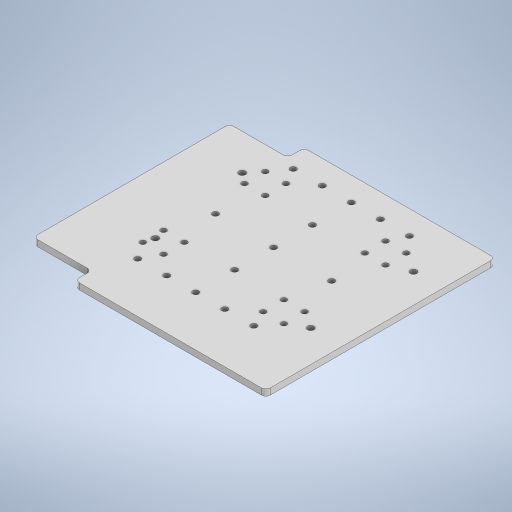
# Autodesk Inventor part: фанера
Saved by Autodesk Inventor 2023 (Build 270158000, 158)
## iProperties
Created: 2025-01-21
Part Number: фанера
Material: Типовые
Document SubType Name: Modeling
Designer: DELL
Density: 1 g/cm^3
Appearance: По умолчанию
Author: DELL
Autodesk Inventor part; units mm, degrees
ref_plane "YZ Plane" through (0, 0, 0) normal (1, 0, 0) x (0, 1, 0)
ref_plane "XZ Plane" through (0, 0, 0) normal (0, 1, 0) x (-1, 0, 0)
ref_plane "XY Plane" through (0, 0, 0) normal (0, 0, 1) x (1, 0, 0)
sketch "Эскиз1" plane through (0, 0, 0) normal (0, 1, 0) x (-1, 0, 0)
  line L0 (-60, 55.25) -> (60, 55.25)
  line L1 (60, 55.25) -> (60, -55.25)
  line L2 (60, -55.25) -> (-60, -55.25)
  line L3 (-60, -55.25) -> (-60, 55.25)
  line L4 (60, -55.25) -> (-60, 55.25) construction
  point P0 (0, 0)
  point P1 (0, 0)
  dimension "d0" = 120
  dimension "d1" = 110.5
  constraints: 10 end point, 2 parallel, 1 coincident, 1 horizontal, 1 midpoint, 1 perpendicular
  measures "d0" distance of L1.end L2.end
  measures "d1" distance of L2.end L0.start
extrude "Выдавливание1" add sketch "Эскиз1" along normal blind 3
sketch "Эскиз2" plane through (0, 3, 0) normal (0, 1, 0) x (1, 0, 0)
  line L0 (-60, 55.25) -> (60, 55.25) projected
  line L1 (-60, 55.25) -> (-32, 55.25)
  line L2 (-32, 55.25) -> (-32, 47.25)
  line L3 (-32, 47.25) -> (-60, 47.25)
  line L4 (-60, 47.25) -> (-60, 55.25)
  line L5 (-60, -55.25) -> (-60, 55.25) projected
  line L6 (-60, -55.25) -> (-32, -55.25)
  line L7 (-32, -55.25) -> (-32, -47.25)
  line L8 (-32, -47.25) -> (-60, -47.25)
  line L9 (-60, -47.25) -> (-60, -55.25)
  point P0 (-60, -47.25)
  dimension "d12" = 28
  dimension "d13" = 8
  dimension "d14" = 28
  dimension "d15" = 8
  constraints: 16 end point, 4 parallel, 2 horizontal, 2 perpendicular
  measures "d12" distance of L2.end L3.end
  measures "d13" distance of L1.end L2.end
  measures "d14" distance of L8.end L7.end
  measures "d15" distance of L7.end L6.end
extrude "Выдавливание2" cut sketch "Эскиз2" against normal blind 10
fillet "Сопряжение2" radius 2 8 edges at (-60, 1.5, 47.25) (-32, 1.5, 47.25) (-32, 1.5, 55.25) (-60, 1.5, -47.25) (-32, 1.5, -47.25) (-32, 1.5, -55.25) (60, 1.5, -55.25) (60, 1.5, 55.25)
sketch "Эскиз3" plane through (0, 3, 0) normal (0, 1, 0) x (1, 0, 0)
  circle A0 centre (-21.5, -13.0622) radius 1.35 projected
  circle A1 centre (-21.5, 35.9378) radius 1.35 projected
  circle A2 centre (36.5, 35.9378) radius 1.35 projected
  circle A3 centre (36.5, -13.0622) radius 1.35 projected
  line L0 (36.5, 25.9378) -> (-21.5, 25.9378) construction
  line L1 (-21.5, 25.9378) -> (-21.5, -23.0622) construction
  line L2 (-21.5, -23.0622) -> (36.5, -23.0622) construction
  line L3 (36.5, -23.0622) -> (36.5, 25.9378) construction
  circle A4 centre (36.5, -23.0622) radius 1.35
  circle A5 centre (36.5, 25.9378) radius 1.35
  circle A6 centre (-21.5, 25.9378) radius 1.35
  circle A7 centre (-21.5, -23.0622) radius 1.35
  line L4 (26.5, 35.9378) -> (-31.5, 35.9378) construction
  line L5 (-31.5, 35.9378) -> (-31.5, -13.0622) construction
  line L6 (-31.5, -13.0622) -> (26.5, -13.0622) construction
  line L7 (26.5, -13.0622) -> (26.5, 35.9378) construction
  circle A8 centre (-31.5, 35.9378) radius 1.35
  circle A9 centre (-31.5, -13.0622) radius 1.35
  circle A10 centre (26.5, -13.0622) radius 1.35
  circle A11 centre (26.5, 35.9378) radius 1.35
  line L8 (26.5, -23.0622) -> (-31.5, -23.0622) construction
  line L9 (-31.5, -23.0622) -> (-31.5, 25.9378) construction
  line L10 (-31.5, 25.9378) -> (26.5, 25.9378)
  line L11 (26.5, 25.9378) -> (26.5, -23.0622) construction
  circle A12 centre (26.5, 25.9378) radius 1.35
  circle A13 centre (26.5, -23.0622) radius 1.35
  circle A14 centre (-31.5, 25.9378) radius 1.35
  circle A15 centre (-31.5, -23.0622) radius 1.35
  point P0 (0, 0)
  dimension "d17" = 58
  dimension "d18" = 49
  dimension "d19" = 10
  dimension "d20" = 58
  dimension "d21" = 49
  dimension "d22" = 10
  dimension "d23" = 2.7
  dimension "d24" = 2.7
  dimension "d25" = 2.7
  dimension "d27" = 58
  dimension "d28" = 49
  dimension "d29" = 2.7
  dimension "d30" = 2.7
  dimension "d31" = 2.7
  dimension "d32" = 2.7
  constraints: 24 end point, 12 centre point, 12 coincident, 6 parallel, 3 horizontal, 3 perpendicular, 2 point on line
  measures "d17" distance of L2.end L1.end
  measures "d18" distance of L1.end L0.end
  measures "d19" distance from line of L0 A2.centre
  measures "d20" distance of L6.end L5.end
  measures "d21" distance of L5.end L4.end
  measures "d22" distance from line of A2.centre L7
  measures "d23" diameter of A8
  measures "d24" diameter of A10
  measures "d25" diameter of A11
  measures "d27" distance of L9.end L10.end
  measures "d28" distance of L8.end L9.end
  measures "d29" diameter of A12
  measures "d30" diameter of A13
  measures "d31" diameter of A14
  measures "d32" diameter of A15
extrude "Выдавливание3" cut sketch "Эскиз3" against normal blind 10
sketch "Эскиз4" plane through (0, 3, 0) normal (0, 1, 0) x (1, 0, 0)
  circle A0 centre (-30.17, -18.3745) radius 1.5875
  circle A1 centre (-36.52, 29.8855) radius 1.5875
  circle A2 centre (46.03, 29.8855) radius 1.5875
  circle A3 centre (44.76, -18.3745) radius 1.5875
  point P0 (0, 0)
  constraints: 4 centre point, 8 other
extrude "Выдавливание4" cut sketch "Эскиз4" against normal blind 10
sketch "Эскиз5" plane through (0, 3, 0) normal (0, 1, 0) x (1, 0, 0)
  point P0 (0, 0)
sketch "Эскиз6" plane through (0, 3, 0) normal (0, 1, 0) x (1, 0, 0)
  circle A0 centre (-25.8393, -31.2041) radius 1.45
  line L0 (-25.8393, -31.2041) -> (2.1607, -31.2041) construction
  line L1 (30.1607, -31.2041) -> (30.1607, 43.7959) construction
  line L2 (30.1607, 43.7959) -> (2.1607, 43.7959) construction
  line L3 (-25.8393, 43.7959) -> (-25.8393, -31.2041) construction
  circle A1 centre (30.1607, -31.2041) radius 1.45
  circle A2 centre (2.1607, -31.2041) radius 1.45
  circle A3 centre (30.1607, 6.2959) radius 1.45
  circle A4 centre (30.1607, 43.7959) radius 1.45
  circle A5 centre (-25.8393, 43.7959) radius 1.45
  circle A6 centre (2.1607, 43.7959) radius 1.45
  circle A7 centre (-25.8393, 6.2959) radius 1.45
  circle A8 centre (2.1607, 6.2959) radius 1.45
  line L4 (2.1607, 43.7959) -> (-25.8393, 43.7959) construction
  line L5 (2.1607, -31.2041) -> (30.1607, -31.2041) construction
  circle A9 centre (16.1607, -31.2041) radius 1.45
  circle A10 centre (-11.8393, -31.2041) radius 1.45
  circle A11 centre (-11.8393, 43.7959) radius 1.45
  circle A12 centre (16.1607, 43.7959) radius 1.45
  line L6 (2.1607, 43.7959) -> (2.1607, 6.2959) construction
  line L7 (2.1607, 6.2959) -> (2.1607, -31.2041) construction
  circle A13 centre (2.1607, -12.4541) radius 1.45
  circle A14 centre (2.1607, 25.0459) radius 1.45
  point P0 (0, 0)
  dimension "d37" = 2.9
  dimension "d38" = 56
  dimension "d39" = 75
  dimension "d40" = 2.9
  dimension "d41" = 2.9
  constraints: 16 end point, 15 centre point, 8 coincident, 8 midpoint, 6 equal length, 2 horizontal, 2 perpendicular, 1 vertical
  measures "d37" diameter of A0
  measures "d38" distance of L3.start L1.end
  measures "d39" distance of L1.end L1.start
  measures "d40" diameter of A1
  measures "d41" diameter of A4
extrude "Выдавливание5" cut sketch "Эскиз6" against normal blind 10
